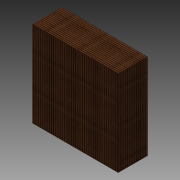
# Autodesk Inventor part: Pièce1
Saved by Autodesk Inventor 2015 (Build 190159000, 159)
## iProperties
Created: 2019-02-09
Part Number: Pièce1
Material: Générique
Document SubType Name: Modeling
Designer: Naly jérémie
Density: 1 g/cm^3
Appearance: Carton
Author: Naly jérémie
Autodesk Inventor part; units mm, degrees
ref_plane "YZ Plane" through (0, 0, 0) normal (1, 0, 0) x (0, 1, 0)
ref_plane "XZ Plane" through (0, 0, 0) normal (0, 1, 0) x (-1, 0, 0)
ref_plane "XY Plane" through (0, 0, 0) normal (0, 0, 1) x (1, 0, 0)
sketch "Esquisse1" plane through (0, 0, 0) normal (0, 1, 0) x (-1, 0, 0)
  line L0 (0, 0) -> (350, 0)
  line L1 (350, 0) -> (350, -350)
  line L2 (350, -350) -> (0, -350)
  line L3 (0, -350) -> (0, 0)
  dimension "d0" = 350
  dimension "d1" = 350
  constraints: 8 end point, 2 parallel, 1 horizontal, 1 perpendicular
  measures "d0" distance of L1.end L2.end
  measures "d1" distance of L0.end L1.end
extrude "Extrusion1" add sketch "Esquisse1" along normal blind 120
sketch "Esquisse2" plane through (0, 120, 0) normal (0, 1, 0) x (1, 0, 0)
  line L0 (0, 350) -> (-350, 350) projected
  line L1 (-350, 350) -> (-350, 0) projected
  circle A0 centre (-175, 175) radius 140
  point P0 (0, 0)
  dimension "d4" = 175
  dimension "d5" = 175
  dimension "d6" = 280
  constraints: 1 centre point, 1 coincident
  measures "d4" distance from line of L0 point (-175, 175)
  measures "d5" distance from line of L1 point (-175, 175)
  measures "d6" diameter of A0
extrude "Extrusion2" cut sketch "Esquisse2" against normal blind 100
